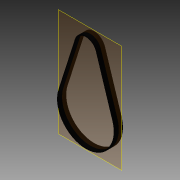
# Autodesk Inventor part: Timming Belt - 165
Saved by Autodesk Inventor 2013 (Build 170138000, 138)
## iProperties
Created: 2013-04-03
Part Number: Timming Belt - 165
Material: Generic
Document SubType Name: Modeling
Designer: mvarma
Density: 1 g/cm^3
Author: mvarma
Autodesk Inventor part; units mm, degrees
ref_plane "YZ Plane" through (0, 0, 0) normal (1, 0, 0) x (0, 1, 0)
ref_plane "XZ Plane" through (0, 0, 0) normal (0, 1, 0) x (-1, 0, 0)
ref_plane "XY Plane" through (0, 0, 0) normal (0, 0, 1) x (1, 0, 0)
sketch "Sketch1" plane through (0, 0, 0) normal (0, 0, 1) x (1, 0, 0)
  arc A0 (0, 30.55) -> (-29.1137, 9.2571) centre (0, 0) ccw construction
  arc A1 (0, 51.5833) -> (10.9117, 66.5028) centre (0, 63.0333) ccw construction
  line L0 (10.9117, 66.5028) -> (29.1137, 9.2571)
  line L1 (-10.9117, 66.5028) -> (-29.1137, 9.2571)
  line L2 (0, 63.0333) -> (0, 0) construction
  arc A2 (-10.9117, 66.5028) -> (0, 51.5833) centre (0, 63.0333) ccw construction
  arc A3 (10.9117, 66.5028) -> (-10.9117, 66.5028) centre (0, 63.0333) ccw
  arc A4 (29.1137, 9.2571) -> (0, 30.55) centre (0, 0) ccw construction
  arc A5 (-29.1137, 9.2571) -> (29.1137, 9.2571) centre (0, 0) ccw
  arc A6 (-11.8647, 66.8058) -> (11.8647, 66.8058) centre (0, 63.0333) ccw construction
  arc A7 (30.0667, 9.5601) -> (-30.0667, 9.5601) centre (0, 0) ccw construction
  line L3 (-11.8647, 66.8058) -> (-30.0667, 9.5601)
  line L4 (11.8647, 66.8058) -> (30.0667, 9.5601)
  arc A8 (11.8647, 66.8058) -> (-11.8647, 66.8058) centre (0, 63.0333) ccw
  arc A9 (-30.0667, 9.5601) -> (30.0667, 9.5601) centre (0, 0) ccw
  dimension "d0" = 60.0698
  dimension "d1" = 22.9
  dimension "d2" = 61.1
  dimension "d3" = 24.9
  dimension "d4" = 63.1
  constraints: 20 point on circle, 12 tangent, 10 centre point, 10 end point, 3 coincident, 2 point on line, 1 vertical
  measures "d0" distance of L0.start L0.end
  measures "d1" diameter of A1
  measures "d2" diameter of A0
  measures "d3" diameter of A6
  measures "d4" diameter of A7
extrude "Extrusion1" add sketch "Sketch1" along normal blind 9
ref_plane "Work Plane1" through (0, 0, 4.5) normal (0, 0, 1) x (1, 0, 0)
body "Solid1"
